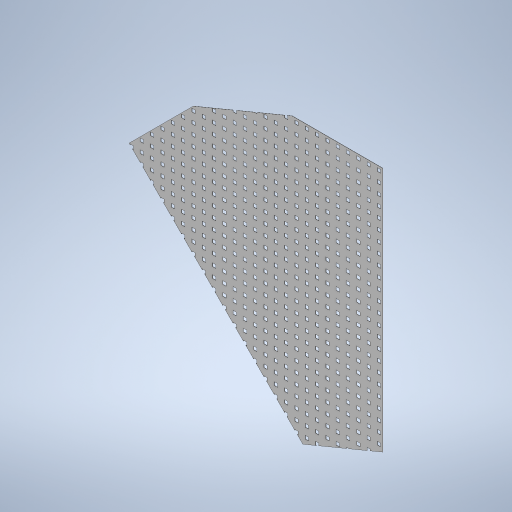
# Autodesk Inventor part: ДМС 207 Сетка кассеты
Saved by Autodesk Inventor 2024.2 (Build 282272000, 272)
## iProperties
Created: 2024-05-05
Part Number: ДМС 207 Сетка кассеты
Material: Generic
Document SubType Name: Sheet Metal
Designer: pokla
Density: 1 g/cm^3
Appearance: Default
Sheet Metal Rule: Default
Author: pokla
Autodesk Inventor part; units mm, degrees
ref_plane "YZ Plane" through (0, 0, 0) normal (1, 0, 0) x (0, 1, 0)
ref_plane "XZ Plane" through (0, 0, 0) normal (0, 1, 0) x (-1, 0, 0)
ref_plane "XY Plane" through (0, 0, 0) normal (0, 0, 1) x (1, 0, 0)
sketch "Sketch1" plane through (0, 0, 0) normal (0, 0, 1) x (1, 0, 0)
  line L0 (0, 273.8452) -> (193.6378, 193.6378) construction
  line L1 (193.6378, 193.6378) -> (273.8452, 0) construction
  line L2 (273.8452, 0) -> (193.6378, -193.6378) construction
  line L3 (193.6378, -193.6378) -> (0, -273.8452) construction
  line L4 (0, -273.8452) -> (-193.6378, -193.6378) construction
  line L5 (-193.6378, -193.6378) -> (-273.8452, 0) construction
  line L6 (-273.8452, 0) -> (-193.6378, 193.6378) construction
  line L7 (-193.6378, 193.6378) -> (0, 273.8452)
  line L8 (-193.6378, 193.6378) -> (0, 273.8452)
  line L9 (-459.9272, 770.6562) -> (-219.7185, 870.1539)
  line L10 (-96.8189, 233.7415) -> (-339.8229, 820.405) construction
  line L11 (-219.7185, 870.1539) -> (0, 870.1539)
  line L12 (0, 870.1539) -> (0, 273.8452)
  line L13 (-459.9272, 770.6562) -> (-615.2917, 615.2917)
  line L14 (-615.2917, 615.2917) -> (-193.6378, 193.6378)
  point P0 (0, 0)
  point P1 (0, 0)
  dimension "d0" = 506
  dimension "d2" = 260
  dimension "d3" = 635
  constraints: 30 end point, 2 midpoint, 1 coincident, 1 horizontal, 1 parallel, 1 perpendicular, 1 symmetric about line, 1 vertical, 1 vertical alignment, 17 other
  measures "d0" distance between parallel lines of L5 L1
  measures "d2" distance of L9.start L9.end
  measures "d3" distance of L10.end L10.start
extrude "Extrusion1" add sketch "Sketch1" along normal mid plane 0.5
sketch "Sketch7" plane through (0, 0, 0.25) normal (0, 0, 1) x (1, 0, 0)
  line L0 (-13, 865.1539) -> (-5, 865.1539)
  line L1 (-5, 865.1539) -> (-5, 857.1539)
  line L2 (-5, 857.1539) -> (-13, 857.1539)
  line L3 (-13, 857.1539) -> (-13, 865.1539)
  line L4 (0, 870.1539) -> (-219.7185, 870.1539) projected
  line L5 (0, 273.8452) -> (0, 870.1539) projected
  point P0 (0, 0)
  dimension "d54" = 8
  dimension "d55" = 8
  dimension "d56" = 5
  dimension "d57" = 5
  constraints: 8 end point, 2 parallel, 1 horizontal, 1 perpendicular
  measures "d54" distance of L1.end L2.end
  measures "d55" distance of L0.end L1.end
  measures "d56" distance between parallel lines of L4 L0
  measures "d57" distance between parallel lines of L5 L1
extrude "Extrusion5" cut sketch "Sketch7" against normal through all
pattern_linear "Rectangular Pattern1" count 30 spacing 25 along (-1, 0, 0) count 30 spacing 25 along (0, -1, 0) of "Extrusion5"
equation "\"d0\" = Барабан_габарит_по_кассетам"
equation "\"d2\" = Кассета_длина_грани"
equation "\"d3\" = Кассета_высота"
equation "\"BendRadius\" = Thickness"
equation "\"BendReliefWidth\" = Thickness"
equation "\"BendReliefDepth\" = 0.5 * Thickness"
equation "\"CornerReliefSize\" = 4 * Thickness"
equation "\"MinimumRemnant\" = 2 * Thickness"
equation "\"TransitionRadius\" = BendRadius"
equation "\"JacobiRadiusSize\" = BendRadius"
equation "\"GapSize\" = Thickness"
equation "\"Барабан_габарит_по_кассетам\" = 506"
equation "\"Кассета_длина_грани\" = 260"
equation "\"Кассета_высота\" = 635"
equation "\"Thickness\" = 0.5"
body "Solid1"
